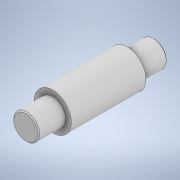
# Autodesk Inventor part: shaft
Saved by Autodesk Inventor 2021 (Build 250183000, 183)
## iProperties
Created: 2022-04-24
Part Number: shaft
Material: Generic
Document SubType Name: Modeling
Designer: hp
Density: 1 g/cm^3
Appearance: Default
Author: hp
Autodesk Inventor part; units mm, degrees
ref_plane "YZ Plane" through (0, 0, 0) normal (1, 0, 0) x (0, 1, 0)
ref_plane "XZ Plane" through (0, 0, 0) normal (0, 1, 0) x (-1, 0, 0)
ref_plane "XY Plane" through (0, 0, 0) normal (0, 0, 1) x (1, 0, 0)
sketch "Sketch1" plane through (0, 0, 0) normal (1, 0, 0) x (0, 1, 0)
  line L0 (21.9008, 5.3079) -> (21.9008, 28.3079)
  line L1 (18.4008, 28.3079) -> (17.6937, 28.3079)
  line L2 (2.4008, 44.015) -> (2.4008, 44.3079)
  line L3 (18.4008, 44.3079) -> (18.4008, 28.3079)
  line L4 (21.9008, 5.3079) -> (17.6937, 5.3079)
  line L5 (3.1079, 44.015) -> (3.1079, 45.015)
  line L6 (10.4008, 45.015) -> (17.6937, 45.015)
  line L7 (17.6937, 44.3079) -> (17.6937, 44.015)
  line L8 (18.4008, 44.3079) -> (17.6937, 45.015)
  line L9 (3.1079, 45.015) -> (2.4008, 44.3079)
  line L10 (21.9008, 5.3079) -> (21.9008, -17.6921)
  line L11 (18.4008, -17.6921) -> (17.6937, -17.6921)
  line L12 (2.4008, -33.3992) -> (2.4008, -33.6921)
  line L13 (18.4008, -33.6921) -> (18.4008, -17.6921)
  line L14 (3.1079, -33.3992) -> (3.1079, -33.6921)
  line L15 (10.4008, -34.3992) -> (17.6937, -34.3992)
  line L16 (18.4008, -33.6921) -> (17.6937, -34.3992)
  line L17 (10.4008, 15) -> (10.4008, -10)
  line L18 (10.4008, 15) -> (10.4008, 87)
  line L19 (10.4008, 87) -> (10.4008, 13)
  line L20 (10.4008, 5.3079) -> (10.4008, -49)
  line L21 (2.4008, 44.3079) -> (3.1079, 44.3079)
  line L22 (17.6937, 44.3079) -> (18.4008, 44.3079)
  line L23 (21.9008, 28.3079) -> (18.4008, 28.3079)
  line L24 (21.9008, -17.6921) -> (18.4008, -17.6921)
  point P0 (0, 0)
  point P1 (0, 10.6157)
  point P2 (3.1079, -34.3992)
  dimension "d1" = 16
  dimension "d2" = 3.5
  dimension "d3" = 23
  dimension "d4" = 16
  dimension "d5" = 1
  dimension "d6" = 1
  dimension "d7" = 11.5
  constraints: 50 end point, 8 point on line, 8 symmetric about line, 4 parallel, 3 horizontal, 2 perpendicular, 2 vertical
  measures "d1" distance between parallel lines of L2 L3
  measures "d2" distance from line of L1.start L0
  measures "d3" distance of L0.start L0.end
  measures "d4" distance of L1.start L3.start
  measures "d5" distance of L3.start L6.end
  measures "d6" distance of L5.end L2.end
  measures "d7" distance between parallel lines of L17 L0
revolve "Revolution1" add sketch "Sketch1" angle 360 about axis through (0, 10.4008, 15) along (0, 0, -1) contours L10 L24 L13 L16 L15 L20 L17 L18 L6 L8 L3 L23 L0
equation "\"d2\" = -0.5 * d1 + 0.5 * d0"
equation "\"d7\" = 0.5 * d0"
equation "\"d0\" = 23"
body "Solid1"
